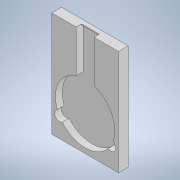
# Autodesk Inventor part: Case Back
Saved by Autodesk Inventor 2022 (Build 260153000, 153)
## iProperties
Created: 2022-10-09
Part Number: Case Back
Material: Generic
Document SubType Name: Modeling
Designer: Nick
Density: 1 g/cm^3
Appearance: Default
Author: Nick
Autodesk Inventor part; units mm, degrees
ref_plane "YZ Plane" through (0, 0, 0) normal (1, 0, 0) x (0, 1, 0)
ref_plane "XZ Plane" through (0, 0, 0) normal (0, 1, 0) x (-1, 0, 0)
ref_plane "XY Plane" through (0, 0, 0) normal (0, 0, 1) x (1, 0, 0)
sketch "Sketch1" plane through (0, 0, 0) normal (0, 0, 1) x (1, 0, 0)
  line L0 (0, 0) -> (68.58, 0)
  line L1 (68.58, 0) -> (68.58, 107.95)
  line L2 (68.58, 107.95) -> (0, 107.95)
  line L3 (0, 107.95) -> (0, 0)
  dimension "d0" = 68.58
  dimension "d1" = 107.95
  constraints: 8 end point, 2 parallel, 1 horizontal, 1 perpendicular
  measures "d0" distance of L2.end L1.end
  measures "d1" distance of L1.end L0.end
extrude "Extrusion1" add sketch "Sketch1" along normal blind 10
sketch "Sketch2" plane through (0, 0, 10) normal (0, 0, 1) x (1, 0, 0)
  circle A0 centre (34.29, 35.56) radius 30.48
  line L0 (0, 0) -> (68.58, 0) projected
  line L1 (68.58, 107.95) -> (0, 107.95) projected
  line L2 (25.1206, 107.95) -> (43.4594, 107.95)
  line L3 (43.4594, 107.95) -> (43.4594, 64.6281)
  line L4 (43.4594, 64.6281) -> (25.1206, 64.6281)
  line L5 (25.1206, 64.6281) -> (25.1206, 107.95)
  circle A1 centre (60.6865, 20.32) radius 5
  circle A2 centre (7.8935, 20.32) radius 5
  line L6 (7.8935, 20.32) -> (34.29, 66.04) construction
  line L7 (34.29, 66.04) -> (60.6865, 20.32) construction
  line L8 (60.6865, 20.32) -> (7.8935, 20.32) construction
  point P0 (34.29, 0)
  point P1 (34.29, 107.95)
  point P2 (57.8397, 16.2095)
  point P3 (62.8229, 24.8406)
  point P4 (10.7403, 16.2095)
  point P5 (5.7571, 24.8406)
  dimension "d4" = 18.3388
  dimension "d5" = 60.96
  dimension "d6" = 35.56
  dimension "d9" = 10
  constraints: 14 end point, 3 centre point, 3 coincident, 3 midpoint, 2 horizontal, 2 parallel, 2 point on circle, 1 equal radius, 1 perpendicular, 1 point on line, 1 vertical alignment, 7 other
  measures "d4" distance of L3.end L4.end
  measures "d5" diameter of A0
  measures "d6" distance from line of L0 A0.centre
  measures "d9" diameter of A2
extrude "Extrusion2" cut sketch "Sketch2" against normal blind 7
sketch "Sketch3" plane through (0, 0, 3) normal (0, 0, 1) x (1, 0, 0)
  arc A0 (25.1206, 64.6281) -> (5.7571, 24.8406) centre (34.29, 35.56) ccw projected
  arc A1 (5.7571, 24.8406) -> (10.7403, 16.2095) centre (7.8935, 20.32) ccw projected
  arc A2 (10.7403, 16.2095) -> (57.8397, 16.2095) centre (34.29, 35.56) ccw projected
  arc A3 (57.8397, 16.2095) -> (62.8229, 24.8406) centre (60.6865, 20.32) ccw projected
  arc A4 (62.8229, 24.8406) -> (43.4594, 64.6281) centre (34.29, 35.56) ccw projected
  line L0 (43.4594, 107.95) -> (43.4594, 64.6281) projected
  line L1 (25.1206, 107.95) -> (43.4594, 107.95) projected
  line L2 (25.1206, 64.6281) -> (25.1206, 107.95) projected
  line L3 (25.1206, 64.6281) -> (25.1206, 107.95) projected
  line L4 (25.1206, 107.95) -> (43.4594, 107.95)
  line L5 (43.4594, 107.95) -> (43.4594, 106.95)
  line L6 (43.4594, 106.95) -> (25.1206, 106.95)
  line L7 (25.1206, 106.95) -> (25.1206, 107.95)
  point P0 (0, 0)
  dimension "d10" = 1
  constraints: 8 end point, 2 parallel, 1 horizontal, 1 perpendicular, 1 point on line
  measures "d10" distance between parallel lines of L1 L6
extrude "Extrusion3" add sketch "Sketch3" along normal blind 1.5 contours L2 L1 L0 L6
body "Solid1"
